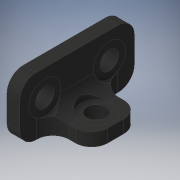
# Autodesk Inventor part: Y Extrusion Bracket
Saved by Autodesk Inventor 2019.4 (Build 234330000, 330)
## iProperties
Created: 2018-06-15
Part Number: Y Extrusion Bracket
Material: ABS Plastic
Document SubType Name: Modeling
Designer: Richard
Density: 1.06 g/cm^3
Appearance: Rubber - Black
Author: Richard
Autodesk Inventor part; units mm, degrees
ref_plane "YZ Plane" through (0, 0, 0) normal (1, 0, 0) x (0, 1, 0)
ref_plane "XZ Plane" through (0, 0, 0) normal (0, 1, 0) x (-1, 0, 0)
ref_plane "XY Plane" through (0, 0, 0) normal (0, 0, 1) x (1, 0, 0)
sketch "Sketch1" plane through (0, 0, 0) normal (1, 0, 0) x (0, 1, 0)
  line L0 (-9, 17.757) -> (9, 17.757)
  line L1 (9, 17.757) -> (9, -17.757)
  line L2 (9, -17.757) -> (-9, -17.757)
  line L3 (-9, -17.757) -> (-9, 17.757)
  line L4 (-9, 17.757) -> (9, -17.757) construction
  line L5 (9, 17.757) -> (-9, -17.757) construction
  circle A0 centre (1, 10) radius 1
  circle A1 centre (1, -10) radius 1
  point P0 (0, 0)
  point P1 (0, 0)
  point P2 (0, 0)
  dimension "d0" = 18
  dimension "d3" = 2
  dimension "d4" = 35.514
  dimension "d28" = 10
  dimension "d29" = 10
  dimension "d30" = 20
  dimension "d31" = 10
  constraints: 12 end point, 4 midpoint, 2 centre point, 2 parallel, 1 equal radius, 1 horizontal, 1 perpendicular
  measures "d0" distance of L1.end L2.end
  measures "d3" diameter of A0
  measures "d4" distance of L0.end L1.end
  measures "d28" distance from line of L3 A1.centre
  measures "d29" distance from line of L3 A0.centre
  measures "d30" distance of A1.centre A0.centre
  measures "d31" vertical distance of A0.centre point (0, 0)
extrude "Extrusion1" add sketch "Sketch1" along normal mid plane 4
sketch "Sketch2" plane through (-2, -9, 12.757) normal (0, -1, 0) x (1, 0, 0)
  line L0 (4, -5.257) -> (16, -5.257)
  line L1 (16, -5.257) -> (16, -20.257)
  line L2 (16, -20.257) -> (4, -20.257)
  line L3 (4, -20.257) -> (4, -5.257)
  line L4 (4, -5.257) -> (16, -20.257) construction
  line L5 (16, -5.257) -> (4, -20.257) construction
  line L6 (4, 5) -> (4, -30.514) projected
  circle A0 centre (10, -12.757) radius 1
  point P0 (-2.0498, -12.757)
  point P1 (10, -12.757)
  point P2 (10, -12.757)
  point P3 (4, -12.757)
  dimension "d8" = 12
  dimension "d9" = 15
  dimension "d13" = 2
  constraints: 12 end point, 5 midpoint, 2 horizontal alignment, 2 parallel, 1 centre point, 1 coincident, 1 collinear, 1 horizontal, 1 perpendicular
  measures "d8" distance of L1.end L2.end
  measures "d9" distance of L0.end L1.end
  measures "d13" diameter of A0
extrude "Extrusion2" add sketch "Sketch2" against normal blind 4
fillet "Fillet2" radius 5 9 edges at (2, -7, 7.5) (2, -5, 0) (2, -7, -7.5) (14, -7, -7.5) (14, -7, 7.5) (0, 9, 17.757) (0, -9, 17.757) (0, 9, -17.757) (0, -9, -17.757)
sketch "Sketch3" plane through (2, 0, 0) normal (1, 0, 0) x (0, 0, -1)
  arc A0 (12.757, -9) -> (17.757, -4) centre (12.757, -4) ccw projected
  line L0 (17.757, -4) -> (17.757, 4) projected
  arc A1 (17.757, 4) -> (12.757, 9) centre (12.757, 4) ccw projected
  line L1 (12.757, 9) -> (-12.757, 9) projected
  arc A2 (-12.757, 9) -> (-17.757, 4) centre (-12.757, 4) ccw projected
  line L2 (-17.757, 4) -> (-17.757, -4) projected
  arc A3 (-17.757, -4) -> (-12.757, -9) centre (-12.757, -4) ccw projected
  line L3 (-12.757, -9) -> (-12.5, -9) projected
  line L4 (-12.5, 0) -> (-12.5, -9) projected
  line L5 (12.5, 0) -> (10, 0) projected
  circle A4 centre (-10, 1) radius 1 projected
  line L6 (10, 0) -> (-10, 0) projected
  circle A5 centre (10, 1) radius 1 projected
  line L7 (-10, 0) -> (-12.5, 0) projected
  line L8 (12.5, -9) -> (12.5, 0) projected
  line L9 (12.5, -9) -> (12.757, -9) projected
  point P0 (0, 0)
  constraints: 2 vertical alignment
hole "Hole1" at (2, 1, 10) at (2, 1, -10) direction (-1, 0, 0) diameter 5.8 end through all start extended yes counterbore diameter 10 counterbore depth 0.001 clearance for "Socket Head Cap Screw" size "M5" standard "Ansi Metric M Profile"
sketch "Sketch4" plane through (-2, -5, 12.757) normal (0, 1, 0) x (1, 0, 0)
  circle A0 centre (10, 12.757) radius 1 projected
  point P0 (2, 12.757)
  point P1 (10, 12.757)
  point P2 (9, 12.757)
  constraints: 1 coincident, 1 horizontal alignment
hole "Hole2" at (8, -5, 0) direction (0, -1, 0) diameter 5.8 end through all start extended yes counterbore diameter 10 counterbore depth 0.001 clearance for "Socket Head Cap Screw" size "M5" standard "Ansi Metric M Profile"
equation "\"d29\" = d28"
equation "\"d31\" = 0.5 * d30"
body "Solid1"
